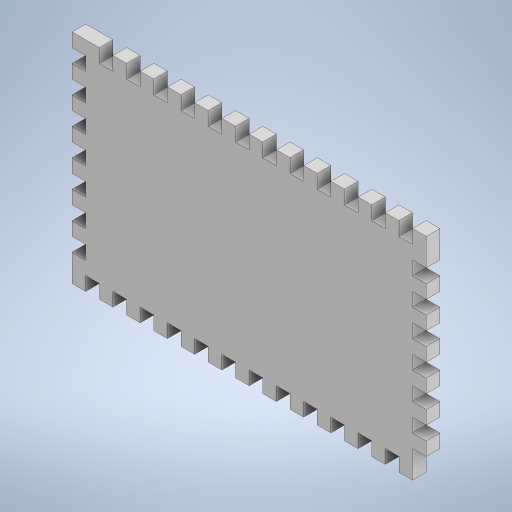
# Autodesk Inventor part: rightside2
Saved by Autodesk Inventor 2024 (Build 280153000, 153)
## iProperties
Created: 2024-04-15
Part Number: rightside2
Material: Generic
Document SubType Name: Modeling
Designer: srika
Density: 1 g/cm^3
Appearance: Default
Author: srika
Autodesk Inventor part; units mm, degrees
ref_plane "YZ Plane" through (0, 0, 0) normal (1, 0, 0) x (0, 1, 0)
ref_plane "XZ Plane" through (0, 0, 0) normal (0, 1, 0) x (-1, 0, 0)
ref_plane "XY Plane" through (0, 0, 0) normal (0, 0, 1) x (1, 0, 0)
sketch "Sketch1" plane through (0, 0, 0) normal (0, 0, 1) x (1, 0, 0)
  line L0 (0, 0) -> (5, 0)
  line L1 (5, 0) -> (5, 5)
  line L2 (5, 5) -> (0, 5)
  line L3 (0, 5) -> (0, 0)
  line L4 (5, 5) -> (125, 5)
  line L5 (125, 5) -> (125, 75)
  line L6 (125, 75) -> (5, 75)
  line L7 (5, 75) -> (5, 5)
  line L8 (130, 80) -> (125, 80)
  line L9 (125, 80) -> (125, 75)
  line L10 (125, 75) -> (130, 75)
  line L11 (130, 75) -> (130, 80)
  line L12 (115, 80) -> (115, 75)
  line L13 (115, 75) -> (120, 75)
  line L14 (120, 75) -> (120, 80)
  line L15 (120, 80) -> (115, 80)
  line L16 (105, 80) -> (105, 75)
  line L17 (105, 75) -> (110, 75)
  line L18 (110, 75) -> (110, 80)
  line L19 (110, 80) -> (105, 80)
  line L20 (95, 80) -> (95, 75)
  line L21 (95, 75) -> (100, 75)
  line L22 (100, 75) -> (100, 80)
  line L23 (100, 80) -> (95, 80)
  line L24 (85, 80) -> (85, 75)
  line L25 (85, 75) -> (90, 75)
  line L26 (90, 75) -> (90, 80)
  line L27 (90, 80) -> (85, 80)
  line L28 (75, 80) -> (75, 75)
  line L29 (75, 75) -> (80, 75)
  line L30 (80, 75) -> (80, 80)
  line L31 (80, 80) -> (75, 80)
  line L32 (65, 80) -> (65, 75)
  line L33 (65, 75) -> (70, 75)
  line L34 (70, 75) -> (70, 80)
  line L35 (70, 80) -> (65, 80)
  line L36 (55, 80) -> (55, 75)
  line L37 (55, 75) -> (60, 75)
  line L38 (60, 75) -> (60, 80)
  line L39 (60, 80) -> (55, 80)
  line L40 (45, 80) -> (45, 75)
  line L41 (45, 75) -> (50, 75)
  line L42 (50, 75) -> (50, 80)
  line L43 (50, 80) -> (45, 80)
  line L44 (35, 80) -> (35, 75)
  line L45 (35, 75) -> (40, 75)
  line L46 (40, 75) -> (40, 80)
  line L47 (40, 80) -> (35, 80)
  line L48 (25, 80) -> (25, 75)
  line L49 (25, 75) -> (30, 75)
  line L50 (30, 75) -> (30, 80)
  line L51 (30, 80) -> (25, 80)
  line L52 (15, 80) -> (15, 75)
  line L53 (15, 75) -> (20, 75)
  line L54 (20, 75) -> (20, 80)
  line L55 (20, 80) -> (15, 80)
  line L56 (5, 80) -> (5, 75)
  line L57 (5, 75) -> (10, 75)
  line L58 (10, 75) -> (10, 80)
  line L59 (10, 80) -> (5, 80)
  line L60 (130, 70) -> (125, 70)
  line L61 (125, 70) -> (125, 75)
  line L62 (125, 75) -> (130, 75)
  line L63 (130, 75) -> (130, 70)
  line L64 (130, 60) -> (125, 60)
  line L65 (125, 60) -> (125, 65)
  line L66 (130, 65) -> (130, 60)
  line L67 (125, 65) -> (130, 65)
  line L68 (125, 65) -> (130, 65)
  line L69 (130, 50) -> (125, 50)
  line L70 (125, 50) -> (125, 55)
  line L71 (130, 55) -> (130, 50)
  line L72 (125, 55) -> (130, 55)
  line L73 (125, 55) -> (130, 55)
  line L74 (130, 40) -> (125, 40)
  line L75 (125, 40) -> (125, 45)
  line L76 (130, 45) -> (130, 40)
  line L77 (125, 45) -> (130, 45)
  line L78 (125, 45) -> (130, 45)
  line L79 (130, 30) -> (125, 30)
  line L80 (125, 30) -> (125, 35)
  line L81 (130, 35) -> (130, 30)
  line L82 (125, 35) -> (130, 35)
  line L83 (125, 35) -> (130, 35)
  line L84 (130, 20) -> (125, 20)
  line L85 (125, 20) -> (125, 25)
  line L86 (130, 25) -> (130, 20)
  line L87 (125, 25) -> (130, 25)
  line L88 (125, 25) -> (130, 25)
  line L89 (130, 10) -> (125, 10)
  line L90 (125, 10) -> (125, 15)
  line L91 (130, 15) -> (130, 10)
  line L92 (125, 15) -> (130, 15)
  line L93 (125, 15) -> (130, 15)
  line L94 (0, 80) -> (5, 80)
  line L95 (5, 80) -> (5, 75)
  line L96 (5, 75) -> (0, 75)
  line L97 (0, 75) -> (0, 80)
  line L98 (5, 70) -> (5, 65)
  line L99 (5, 65) -> (0, 65)
  line L100 (0, 70) -> (5, 70)
  line L101 (0, 65) -> (0, 70)
  line L102 (5, 70) -> (5, 65)
  line L103 (5, 60) -> (5, 55)
  line L104 (5, 55) -> (0, 55)
  line L105 (0, 60) -> (5, 60)
  line L106 (0, 55) -> (0, 60)
  line L107 (5, 60) -> (5, 55)
  line L108 (5, 50) -> (5, 45)
  line L109 (5, 45) -> (0, 45)
  line L110 (0, 50) -> (5, 50)
  line L111 (0, 45) -> (0, 50)
  line L112 (5, 50) -> (5, 45)
  line L113 (5, 40) -> (5, 35)
  line L114 (5, 35) -> (0, 35)
  line L115 (0, 40) -> (5, 40)
  line L116 (0, 35) -> (0, 40)
  line L117 (5, 40) -> (5, 35)
  line L118 (5, 30) -> (5, 25)
  line L119 (5, 25) -> (0, 25)
  line L120 (0, 30) -> (5, 30)
  line L121 (0, 25) -> (0, 30)
  line L122 (5, 30) -> (5, 25)
  line L123 (5, 20) -> (5, 15)
  line L124 (5, 15) -> (0, 15)
  line L125 (0, 20) -> (5, 20)
  line L126 (0, 15) -> (0, 20)
  line L127 (5, 20) -> (5, 15)
  line L128 (5, 10) -> (5, 5)
  line L129 (5, 5) -> (0, 5)
  line L130 (0, 10) -> (5, 10)
  line L131 (0, 5) -> (0, 10)
  line L132 (5, 10) -> (5, 5)
  line L133 (125, 30) -> (90, 30)
  line L134 (90, 30) -> (90, 5)
  line L135 (10, 0) -> (15, 0)
  line L136 (15, 0) -> (15, 5)
  line L137 (10, 5) -> (10, 0)
  line L138 (20, 0) -> (25, 0)
  line L139 (25, 0) -> (25, 5)
  line L140 (20, 5) -> (20, 0)
  line L141 (30, 0) -> (35, 0)
  line L142 (35, 0) -> (35, 5)
  line L143 (30, 5) -> (30, 0)
  line L144 (40, 0) -> (45, 0)
  line L145 (45, 0) -> (45, 5)
  line L146 (40, 5) -> (40, 0)
  line L147 (50, 0) -> (55, 0)
  line L148 (55, 0) -> (55, 5)
  line L149 (50, 5) -> (50, 0)
  line L150 (60, 0) -> (65, 0)
  line L151 (65, 0) -> (65, 5)
  line L152 (60, 5) -> (60, 0)
  line L153 (70, 0) -> (75, 0)
  line L154 (75, 0) -> (75, 5)
  line L155 (70, 5) -> (70, 0)
  line L156 (80, 0) -> (85, 0)
  line L157 (85, 0) -> (85, 5)
  line L158 (80, 5) -> (80, 0)
  line L159 (90, 0) -> (95, 0)
  line L160 (95, 0) -> (95, 5)
  line L161 (90, 5) -> (90, 0)
  line L162 (100, 0) -> (105, 0)
  line L163 (105, 0) -> (105, 5)
  line L164 (100, 5) -> (100, 0)
  line L165 (110, 0) -> (115, 0)
  line L166 (115, 0) -> (115, 5)
  line L167 (110, 5) -> (110, 0)
  line L168 (120, 0) -> (125, 0)
  line L169 (125, 0) -> (125, 5)
  line L170 (120, 5) -> (120, 0)
  point P0 (5, 65)
  point P1 (5, 55)
  point P2 (5, 45)
  point P3 (5, 35)
  point P4 (5, 25)
  point P5 (5, 15)
  point P6 (5, 5)
  dimension "d2" = 120
  dimension "d36" = 70
  dimension "d53" = 10
  dimension "d60" = 10
  dimension "d67" = 10
  dimension "d74" = 10
  constraints: 338 end point, 96 horizontal alignment, 57 parallel, 36 collinear, 5 horizontal, 4 perpendicular, 4 vertical, 144 other
  measures "d2" distance of L7.start L5.end
  measures "d36" distance of L5.start L5.end
  measures "d53" distance of L5.end L12.end
  measures "d60" distance of L5.end L65.end
  measures "d67" distance of L7.start point (5, 65)
  measures "d74" distance of L0.start L135.start
extrude "Extrusion2" add sketch "Sketch1" along normal blind 5
body "Solid2"
